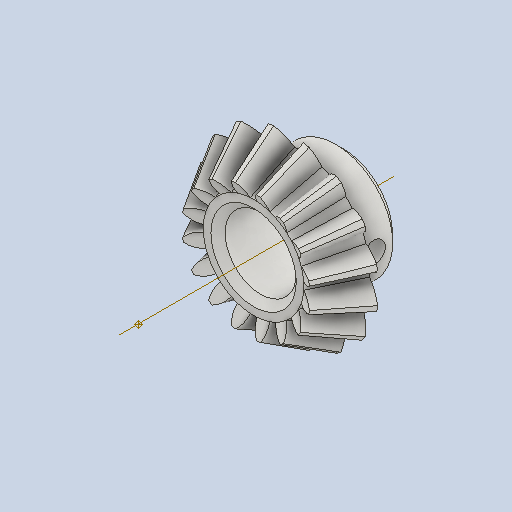
# Autodesk Inventor part: KisKupkerek
Saved by Autodesk Inventor 2023.3 (Build 273359000, 359)
## iProperties
CustomPartVersion: 1
Created: 2023-11-24
Part Number: KisKupkerek
Material: Steel, Mild
Document SubType Name: Modeling
Designer: Csábi-Kis Henrik
Categories: <?xml version="1.0" encoding="UTF-16"?> <MemberInstance><Categories><FamilyTemplate><FamilyTemplateParameter ValueType="xs:double" Id="1" ObjectReferenceKey="da_z" ObjectType="kUserParameterObject"/><FamilyTemplateParameter ValueType="xs:double" Id="2" ObjectReferenceKey="da_b" ObjectType="kUserParameterObject"/><FamilyTemplateParameter ValueType="xs:double" Id="3" ObjectReferenceKey="da_beta" ObjectType="kUserParameterObject"/><FamilyTemplateParameter ValueType="xs:double" Id="4" ObjectReferenceKey="da_dae" ObjectType="kUserParameterObject"/><FamilyTemplateParameter ValueType="xs:double" Id="5" ObjectReferenceKey="da_ve" ObjectType="kUserParameterObject"/><FamilyTemplateParameter ValueType="xs:double" Id="6" ObjectReferenceKey="da_omega" ObjectType="kUserParameterObject"/><FamilyTemplateParameter ValueType="xs:string" Id="7" ObjectReferenceKey="EAIAABAAAAAAHwAAAAAAAIAAAAAAAAAA" ObjectType="83914240" SubObjectId="SurfaceGeometry"/></FamilyTemplate><ParamToTemplateMap><ParamToTemplate CategoryParameter="//CategoryParameter[@InternalName='046C89C9-8512-4d59-83FE-43B91F4F132A']" TemplateParameter="1"/><ParamToTemplate CategoryParameter="//CategoryParameter[@InternalName='2552DF32-E462-4b46-AEBF-C6C7768E72AC']" TemplateParameter="2"/><ParamToTemplate CategoryParameter="//CategoryParameter[@InternalName='C9EE641D-15FC-4fae-A226-E94C4372FDD7']" TemplateParameter="3"/><ParamToTemplate><ParamToTemplate CategoryParameter="//CategoryParameter[@InternalName='00B6519A-459B-49c7-AD84-2E56D39A5744']" ConstantValue="-0.000000"/></ParamToTemplate><ParamToTemplate><ParamToTemplate CategoryParameter="//CategoryParameter[@InternalName='04B31F0E-C7A6-4894-AA32-9629BEFACF47']" ConstantValue="1.000000"/></ParamToTemplate><ParamToTemplate><ParamToTemplate CategoryParameter="//CategoryParameter[@InternalName='43CBEC2E-7847-49e7-A936-2F7889FCB2D9']" ConstantValue="0.200000"/></ParamToTemplate><ParamToTemplate><ParamToTemplate CategoryParameter="//CategoryParameter[@InternalName='B1EFC894-105D-4ebd-86BF-FA20ED196853']" ConstantValue="0.300000"/></ParamToTemplate><ParamToTemplate><ParamToTemplate CategoryParameter="//CategoryParameter[@InternalName='51175063-3D10-4879-93E8-6246FE8B403D']" ConstantValue="2060000000.000000"/></ParamToTemplate><ParamToTemplate><ParamToTemplate CategoryParameter="//CategoryParameter[@InternalName='A3A52E27-4454-46a9-B0BD-C932399B70AF']" ConstantValue="0.300000"/></ParamToTemplate><ParamToTemplate CategoryParameter="//CategoryParameter[@InternalName='2A200944-5A8C-41ca-B96E-8520D2E510F1']" TemplateParameter="4"/><ParamToTemplate><ParamToTemplate CategoryParameter="//CategoryParameter[@InternalName='1A637F62-92C8-44bc-B81F-10802510B579']" ConstantValue="1.808865"/></ParamToTemplate><ParamToTemplate CategoryParameter="//CategoryParameter[@InternalName='B52DD4BE-6863-48fb-BF58-89EF6F9EC65C']" TemplateParameter="5"/><ParamToTemplate><ParamToTemplate CategoryParameter="//CategoryParameter[@InternalName='3956BFF2-84D2-457d-93C2-9B0613DEBA67']" ConstantValue="1.479436"/></ParamToTemplate><ParamToTemplate CategoryParameter="//CategoryParameter[@InternalName='739CFA02-461B-4bf8-8049-181FCAD8B28F']" TemplateParameter="6"/><ParamToTemplate><ParamToTemplate CategoryParameter="//CategoryParameter[@InternalName='A27E999F-E2CE-4481-8A2A-EBF499C4C3C5']" ConstantValue="-0.000000"/></ParamToTemplate><ParamToTemplate><ParamToTemplate CategoryParameter="//CategoryParameter[@InternalName='9E1B4470-B2D3-4ff1-B813-535BB4CDF51A']" ConstantValue="3520000.000000"/></ParamToTemplate><ParamToTemplate><ParamToTemplate CategoryParameter="//CategoryParameter[@InternalName='F8452263-BFF6-458c-9FB1-07C4B99E95CD']" ConstantValue="11400000.000000"/></ParamToTemplate><ParamToTemplate><ParamToTemplate CategoryParameter="//CategoryParameter[@InternalName='3E3BB259-FD49-497f-8171-6EBC954A3479']" ConstantValue="2.000000"/></ParamToTemplate><ParamToTemplate CategoryParameter="//CategoryParameter[@InternalName='27C3BAF2-7550-4e4b-AE2C-0DB134B7D9B7']" TemplateParameter="7"/></ParamToTemplateMap><Category DisplayName="Gear" InternalName="DC85795E-93AB-48d5-8EEE-5A27447B64BD" Mnemonic="Gear"><CategoryParameter DisplayName="z" InternalName="046C89C9-8512-4d59-83FE-43B91F4F132A" Mnemonic="z"/><CategoryParameter DisplayName="b" InternalName="2552DF32-E462-4b46-AEBF-C6C7768E72AC" Mnemonic="b"/><CategoryParameter DisplayName="||b|" InternalName="C9EE641D-15FC-4fae-A226-E94C4372FDD7" Mnemonic="beta"/><CategoryParameter DisplayName="x" InternalName="00B6519A-459B-49c7-AD84-2E56D39A5744" Mnemonic="x"/><CategoryParameter DisplayName="a*" InternalName="04B31F0E-C7A6-4894-AA32-9629BEFACF47" Mnemonic="a"/><CategoryParameter DisplayName="c*" InternalName="43CBEC2E-7847-49e7-A936-2F7889FCB2D9" Mnemonic="c"/><CategoryParameter DisplayName="r|.f|*" InternalName="B1EFC894-105D-4ebd-86BF-FA20ED196853" Mnemonic="rf"/><CategoryParameter DisplayName="E" InternalName="51175063-3D10-4879-93E8-6246FE8B403D" Mnemonic="E"/><CategoryParameter DisplayName="||m|" InternalName="A3A52E27-4454-46a9-B0BD-C932399B70AF" Mnemonic="mi"/><Category DisplayName="BevelGear" InternalName="0C98F69A-0C2B-4791-B2FE-7691BB227E77" Mnemonic="BevelGear"><CategoryParameter DisplayName="d|.ae|" InternalName="2A200944-5A8C-41ca-B96E-8520D2E510F1" Mnemonic="dae"/><CategoryParameter DisplayName="d|.ai|" InternalName="1A637F62-92C8-44bc-B81F-10802510B579" Mnemonic="dai"/><CategoryParameter DisplayName="A|.e|" InternalName="B52DD4BE-6863-48fb-BF58-89EF6F9EC65C" Mnemonic="ve"/><CategoryParameter DisplayName="A|.i|" InternalName="3956BFF2-84D2-457d-93C2-9B0613DEBA67" Mnemonic="vi"/><CategoryParameter DisplayName="||S|" InternalName="739CFA02-461B-4bf8-8049-181FCAD8B28F" Mnemonic="omega"/><CategoryParameter DisplayName="x|.t|" InternalName="A27E999F-E2CE-4481-8A2A-EBF499C4C3C5" Mnemonic="xt"/><CategoryParameter DisplayName="||s||.Flim|" InternalName="9E1B4470-B2D3-4ff1-B813-535BB4CDF51A" Mnemonic="sFlim"/><CategoryParameter DisplayName="||s||.Hlim|" InternalName="F8452263-BFF6-458c-9FB1-07C4B99E95CD" Mnemonic="sHlim"/><CategoryParameter DisplayName="type" InternalName="3E3BB259-FD49-497f-8171-6EBC954A3479" Mnemonic="type"/><CategoryParameter DisplayName="PitchDiameter" InternalName="27C3BAF2-7550-4e4b-AE2C-0DB134B7D9B7" Mnemonic="IDS_PITCHDIAM"/></Category></Category></Categories></MemberInstance>
Mass: 17.0865 g
Surface Area: 20.0038 cm^2
Volume: 2.17663 cm^3
Density: 7.85 g/cm^3
Appearance: Steel
Author: Csábi-Kis Henrik
Autodesk Inventor part; units mm, degrees
ref_plane "Mesh Plane2" through (0, 0, 0) normal (0.9807853, 0.1950903, 0) x (0, 0, 1)
sketch "Teeth Body Sketch" plane through (0, 0, 0) normal (1, 0, 0) x (0, 1, 0)
  line L0 (0, 0) -> (9.9259, -22.2575) construction
  line L1 (9.9259, -22.2575) -> (12.7018, -20.7771)
  line L2 (12.7018, -20.7771) -> (0, 0) construction
  line L3 (11.44, -21.45) -> (0, 0) construction
  line L4 (7.0678, -15.8485) -> (9.0443, -14.7944)
  line L5 (9.9259, -22.2575) -> (7.0678, -15.8485)
  line L6 (12.7018, -20.7771) -> (9.0443, -14.7944)
  line L7 (0, -26.709) -> (0, 4.4515) projected
  line L8 (0, -21.45) -> (12.7018, -21.45) construction
  dimension "d0" = 22.88
  dimension "d1" = 19.8518
  dimension "d2" = 25.4035
  dimension "d3" = 7
  dimension "d4" = 20.7771
  constraints: 16 end point, 4 point on line, 3 perpendicular, 2 collinear, 1 horizontal alignment, 1 vertical alignment
  measures "d0" diameter of L3.start L7
  measures "d1" diameter of L0.end L7
  measures "d2" diameter of L1.end L7
  measures "d3" distance between parallel lines of L1 L4
  measures "d4" vertical distance of L1.end L0.start
revolve "Teeth Body" add sketch "Teeth Body Sketch" angle 360 about axis through (0, 0, 0) along (0, 0, 1)
ref_plane "Tooth Plane" through (0, 11.44, -21.45) normal (0, -0.4705882, 0.8823529) x (1, 0, 0)
sketch "Start Sketch" plane through (0, 11.44, -21.45) normal (0, -0.4705882, 0.8823529) x (1, 0, 0)
  line L0 (0, -16.0344) -> (0, 5.4493) projected
  arc A0 (-0.6387, -2.0935) -> (-3.1013, 2.057) centre (-5.5511, -2.2023) ccw
  arc A1 (3.1013, 2.057) -> (0.6387, -2.0935) centre (5.5511, -2.2023) ccw
  line L1 (-0.6387, -2.0935) -> (0.6387, -2.0935)
  arc A2 (3.1013, 2.057) -> (-3.1013, 2.057) centre (0, -12.9653) ccw
  dimension "d7" = 4.9136
  dimension "d8" = 5.5511
  dimension "d9" = 10.763
  dimension "d57" = 15.3391
  dimension "d58" = 10.8718
  constraints: 6 point on circle, 3 centre point, 3 symmetric about line, 2 end point, 1 coincident, 1 perpendicular, 1 other
  measures "d7" radius of A0
  measures "d8" horizontal distance of point (0, -12.965) A0.centre
  measures "d9" vertical distance of point (0, -12.965) A0.centre
  measures "d57" radius of A2
  measures "d58" distance from line of A2.centre L1
sketch "End Sketch" plane through (0, 8.0719, -15.1347) normal (0, -0.4705882, 0.8823529) x (1, 0, 0)
  line L0 (0, -10.654) -> (0, 3.6208) projected
  arc A0 (-0.4507, -1.4772) -> (-2.1883, 1.4514) centre (-3.9167, -1.5539) ccw
  arc A1 (2.1883, 1.4514) -> (0.4507, -1.4772) centre (3.9167, -1.5539) ccw
  line L1 (-0.4507, -1.4772) -> (0.4507, -1.4772)
  arc A2 (2.1883, 1.4514) -> (-2.1883, 1.4514) centre (0, -9.1481) ccw
  dimension "d12" = 3.4669
  dimension "d15" = 3.9167
  dimension "d16" = 7.5942
  dimension "d59" = 10.823
  dimension "d60" = 7.671
  constraints: 6 point on circle, 3 centre point, 3 symmetric about line, 2 end point, 1 coincident, 1 other
  measures "d12" radius of A0
  measures "d15" horizontal distance of A0.centre point (0, -9.148)
  measures "d16" vertical distance of A0.centre point (0, -9.148)
  measures "d59" radius of A2
  measures "d60" distance from line of A2.centre L1
loft "Loft" cut profiles "Start Sketch", "End Sketch"
pattern_circular "Circular Pattern" count 16 over 360 about axis through (0, 0, 0) along (0, 0, 1) of "Loft"
ref_plane "End Plane" through (0, 8.0719, -15.1347) normal (0, -0.4705882, 0.8823529) x (1, 0, 0)
sketch3d "3D Sketch Right"
ref_plane "End Plane Right" through (-2.4304, 7.6973, -15.1347) normal (0.1416918, -0.4487502, 0.8823529) x (0.9535941, 0.3010951, 0)
sketch "End Sketch Right" plane through (-2.4304, 7.6973, -15.1347) normal (0.1416918, -0.4487502, 0.8823529) x (0.9535941, 0.3010951, 0)
  arc A0 (-0.4507, -1.4772) -> (-2.1883, 1.4514) centre (-3.9167, -1.5539) ccw
  line L0 (0, -13.9104) -> (0, 6.3438) projected
  arc A1 (2.1883, 1.4514) -> (0.4507, -1.4772) centre (3.9167, -1.5539) ccw
  line L1 (-0.4507, -1.4772) -> (0.4507, -1.4772)
  arc A2 (2.1883, 1.4514) -> (-2.1883, 1.4514) centre (0, -9.1481) ccw
  dimension "d70" = 3.9167
  dimension "d71" = 7.5942
  dimension "d72" = 3.4669
  dimension "d73" = 7.671
  dimension "d74" = 10.823
  constraints: 6 point on circle, 3 centre point, 3 symmetric about line, 2 end point, 1 coincident, 1 perpendicular, 1 other
  measures "d70" horizontal distance of A2.centre A0.centre
  measures "d71" vertical distance of point (0, -9.148) A0.centre
  measures "d72" radius of A0
  measures "d73" distance from line of point (0, -9.148) L1
  measures "d74" radius of A2
feature "Loft Right" [suppressed]
pattern_circular "Circular Pattern Right" [suppressed]
sketch3d "3D Sketch Left"
ref_plane "End Plane Left" through (2.4199, 7.6973, -15.1307) normal (-0.1411215, -0.448882, 0.8823773) x (0.9539668, -0.2999123, 0)
sketch "End Sketch Left" plane through (2.4199, 7.6973, -15.1307) normal (-0.1411215, -0.448882, 0.8823773) x (0.9539668, -0.2999123, 0)
  line L0 (0, -23.2336) -> (0, 10.7413) projected
  arc A0 (-0.4507, -1.4763) -> (-2.1883, 1.4523) centre (-3.9167, -1.553) ccw
  arc A1 (2.1883, 1.4523) -> (0.4507, -1.4763) centre (3.9167, -1.553) ccw
  line L1 (-0.4507, -1.4763) -> (0.4507, -1.4763)
  ellipse E0 centre (0, -6.9614) end of major axis (9.0443, -6.9614) minor radius 7.9805 projected
  arc A2 (2.1883, 1.4523) -> (-2.1883, 1.4523) centre (0, -9.1472) ccw
  dimension "d56" = 7.9805
  dimension "d30" = 3.4669
  dimension "d31" = 3.9167
  dimension "d32" = 7.5942
  dimension "d61" = 10.823
  dimension "d62" = 7.671
  constraints: 6 point on circle, 3 centre point, 3 symmetric about line, 2 end point, 1 coincident, 2 other
  measures "d30" radius of A0
  measures "d31" horizontal distance of point (0, -9.147) A0.centre
  measures "d32" vertical distance of A0.centre point (0, -9.147)
  measures "d61" radius of A2
  measures "d62" distance from line of point (0, -9.147) L1
feature "Loft Left" [suppressed]
pattern_circular "Circular Pattern Left" [suppressed]
sketch "Body Sketch" plane through (0, 0, 0) normal (1, 0, 0) x (0, 1, 0)
  line L0 (0, -23.7224) -> (0, -13.468) projected
  line L1 (9.9259, -22.2575) -> (7.0678, -15.8485) projected
  line L2 (7.0678, -15.8485) -> (0, -15.8485)
  line L3 (9.9259, -22.2575) -> (0, -22.2575)
  constraints: 4 end point, 2 perpendicular, 2 point on line
revolve "Fix Body" add sketch "Body Sketch" angle 360 about axis through (0, 0, 0) along (0, 0, 1)
sketch "Sketch6" plane through (0, 0, 0) normal (1, 0, 0) x (0, 1, 0)
  line L0 (11.44, -21.45) -> (0, 0) projected
  line L1 (0, -25.74) -> (0, 4.29) projected
surface revolve "Pitch Diameter" sketch "Sketch6" angle 360 about axis through (0, 0, 0) along (0, 0, 1) shown no curves L0
sketch "Sketch8" plane through (0, 0, -22.2575) normal (0, 0, -1) x (-1, 0, 0)
  circle A0 centre (0, 0) radius 8
  dimension "d94" = 16
  constraints: 1 centre point, 1 coincident
  measures "d94" diameter of A0
extrude "Extrusion1" add sketch "Sketch8" along normal blind 6.142
sketch "Sketch9" plane through (0, 0, -15.8485) normal (0, 0, 1) x (1, 0, 0)
  point P0 (0, 0)
hole "Hole1" at (0, 0, -15.8485) direction (0, 0, -1) diameter 10 end through all
sketch "Sketch10" plane through (0, 0, 0) normal (1, 0, 0) x (0, 1, 0)
  line L0 (0, 5.6799) -> (0, -34.0794) projected
  line L1 (8, -22.2575) -> (-8, -22.2575) projected
  point P0 (0, -24.8995)
  dimension "d104" = 2.642
  constraints: 1 point on line
  measures "d104" distance from line of L1 point (0, -24.9)
hole "Hole2" at (0, 0, -24.8995) direction (-1, 0, 0) diameter 3 end through all both
chamfer "Chamfer1" distance 1 angle 45 2 edges at (8, 0, -28.3995) (0, 5, -15.8485)
chamfer "Chamfer2" distance 0.5 angle 45 1 edges at (0, 5, -28.3995)
equation "\"d0\" = da_de"
equation "\"d1\" = da_dfe"
equation "\"d2\" = da_dae"
equation "\"d3\" = da_b"
equation "\"d4\" = da_ve"
equation "\"d7\" = fd_rr"
equation "\"d8\" = fd_x"
equation "\"d9\" = fd_y"
equation "\"d57\" = 0.5 * fd_dva + 0.3 * da_he"
equation "\"d58\" = 0.5 * fd_dva - 1.12 * da_he"
equation "\"da_teethtype\" = 0"
equation "\"d97\" = FuroTengelyAtmero"
equation "\"d105\" = SzegAtmero"
equation "\"da_b\" = 7"
equation "\"da_de\" = 22.88"
equation "\"da_dae\" = 25.40353"
equation "\"da_dfe\" = 19.85176"
equation "\"da_le\" = 24.31"
equation "\"da_omega\" = 90deg"
equation "\"da_beta\" = 0"
equation "\"da_delta\" = 28.072487deg"
equation "\"da_alpha\" = 20deg"
equation "\"da_he\" = 3.146"
equation "\"da_ve\" = 20.77706"
equation "\"da_zv\" = 18.133333"
equation "\"fd_loft\" = da_b + 0.05 * da_he"
equation "\"fd_x\" = fd_x1 + fd_x2"
equation "\"fd_y\" = fd_y1 - fd_y2"
equation "\"fd_dd\" = fd_dva - 0.8 * da_he"
equation "\"da_dvw\" = 25.93067"
equation "\"d11\" = fd_loft"
equation "\"da_dm\" = 19.58588"
equation "\"da_x\" = 0"
equation "\"da_m\" = 1.43"
equation "\"d50\" = da_omega"
equation "\"fd_rr\" = 4.913563"
equation "\"fd_dva\" = 28.790667"
equation "\"FuroTengelyAtmero\" = 10"
equation "\"SzegAtmero\" = 3"
equation "\"fd_x1\" = 1.134147"
equation "\"fd_x2\" = 4.416937"
equation "\"fd_y1\" = 12.915633"
equation "\"fd_y2\" = 2.152619"
body "Solid1"
body "Srf1"
